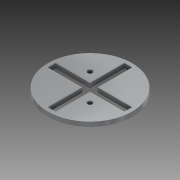
# Autodesk Inventor part: TransparentTop
Saved by Autodesk Inventor 2014 (Build 180170000, 170)
## iProperties
Created: 2013-12-17
Part Number: TransparentTop
Material: Generic
Document SubType Name: Modeling
Designer: blacki
Density: 1 g/cm^3
Appearance: Clear Reflective
Author: blacki
Autodesk Inventor part; units mm, degrees
ref_plane "YZ Plane" through (0, 0, 0) normal (1, 0, 0) x (0, 1, 0)
ref_plane "XZ Plane" through (0, 0, 0) normal (0, 1, 0) x (-1, 0, 0)
ref_plane "XY Plane" through (0, 0, 0) normal (0, 0, 1) x (1, 0, 0)
sketch "Sketch1" plane through (0, 0, 0) normal (0, 0, 1) x (1, 0, 0)
  circle A0 centre (0, 0) radius 27.5
  dimension "d0" = 55
  constraints: 1 centre point, 1 coincident
  measures "d0" diameter of A0
extrude "Extrusion1" add sketch "Sketch1" along normal blind 3
sketch "Sketch2" plane through (0, 0, 0) normal (0, 0, -1) x (-1, 0, 0)
  circle A0 centre (0, 0) radius 27.5 projected
  line L0 (-2.5, -25) -> (-2.5, 25)
  line L1 (-2.5, 25) -> (2.5, 25)
  line L2 (2.5, 25) -> (2.5, -25)
  line L3 (2.5, -25) -> (-2.5, -25)
  line L4 (-2.5, -25) -> (2.5, 25) construction
  line L5 (-2.5, 25) -> (2.5, -25) construction
  line L6 (-25, -2.5) -> (25, -2.5)
  line L7 (25, -2.5) -> (25, 2.5)
  line L8 (25, 2.5) -> (-25, 2.5)
  line L9 (-25, 2.5) -> (-25, -2.5)
  line L10 (-25, -2.5) -> (25, 2.5) construction
  line L11 (25, -2.5) -> (-25, 2.5) construction
  dimension "d3" = 50
  dimension "d4" = 5
  dimension "d5" = 50
  dimension "d6" = 5
  constraints: 24 end point, 4 midpoint, 4 parallel, 2 perpendicular, 1 horizontal, 1 vertical
  measures "d3" distance between parallel lines of L3 L1
  measures "d4" distance between parallel lines of L2 L0
  measures "d5" distance of L8.end L7.end
  measures "d6" distance of L7.end L6.end
extrude "Extrusion2" cut sketch "Sketch2" against normal up to next contours L0 L6 L2 L3 | L6 L9 L8 L0 | L0 L8 L2 L6 | L0 L1 L2 L8 | L2 L8 L7 L6
sketch "Sketch3" plane through (0, 0, 0) normal (0, 0, -1) x (-1, 0, 0)
  circle A0 centre (8.8388, 8.8388) radius 1.5 projected
  circle A1 centre (-8.8388, -8.8388) radius 1.5 projected
extrude "Extrusion3" cut sketch "Sketch3" against normal up to next
body "Solid1"
